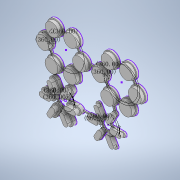
# Autodesk Inventor part: button_all
Saved by Autodesk Inventor 2022 (Build 260153000, 153)
## iProperties
Created: 2022-07-05
Part Number: button_all
Material: 常规
Document SubType Name: Modeling
Designer: yangmc
Density: 1 g/cm^3
Appearance: 默认
Author: yangmc
Autodesk Inventor part; units mm, degrees
ref_plane "YZ Plane" through (0, 0, 0) normal (1, 0, 0) x (0, 1, 0)
ref_plane "XZ Plane" through (0, 0, 0) normal (0, 1, 0) x (-1, 0, 0)
ref_plane "XY Plane" through (0, 0, 0) normal (0, 0, 1) x (1, 0, 0)
sketch "草图1" plane through (0, 0, 0) normal (0, 0, 1) x (1, 0, 0)
  line L0 (24.3527, -0.0988) -> (30.3527, -0.0988) construction
  line L1 (24.3527, -1.5988) -> (30.3527, -1.5988)
  line L2 (30.3527, 1.4012) -> (24.3527, 1.4012)
  arc A0 (24.3527, 1.4012) -> (24.3527, -1.5988) centre (24.3527, -0.0988) ccw
  arc A1 (30.3527, -1.5988) -> (30.3527, 1.4012) centre (30.3527, -0.0988) ccw
  line L3 (25.3527, -0.0988) -> (29.3527, -0.0988) construction
  line L4 (25.3527, -1.5988) -> (29.3527, -1.5988)
  line L5 (29.3527, 1.4012) -> (25.3527, 1.4012)
  arc A2 (25.3527, 1.4012) -> (25.3527, -1.5988) centre (25.3527, -0.0988) ccw
  arc A3 (29.3527, -1.5988) -> (29.3527, 1.4012) centre (29.3527, -0.0988) ccw
  circle A4 centre (-2.7903, 26.7021) radius 4.75
  circle A5 centre (-2.7903, 26.7021) radius 4
  line L6 (-3, 0) -> (3, 0) construction
  line L7 (-2, 0) -> (2, 0) construction
  line L8 (-2, -1.5) -> (2, -1.5)
  line L9 (2, 1.5) -> (-2, 1.5)
  arc A6 (-2, 1.5) -> (-2, -1.5) centre (-2, 0) ccw
  arc A7 (2, -1.5) -> (2, 1.5) centre (2, 0) ccw
  line L10 (-4.5, 0) -> (4.5, 0) construction
  line L11 (-2, -2.5) -> (2, -2.5)
  line L12 (2, 2.5) -> (-2, 2.5)
  arc A8 (-2, 2.5) -> (-2, -2.5) centre (-2, 0) ccw
  arc A9 (2, -2.5) -> (2, 2.5) centre (2, 0) ccw
  circle A10 centre (7.733, 0) radius 1.0239
  arc A11 (6.1655, -5.7149) -> (3.5674, -4.2149) centre (4.8665, -4.9649) ccw
  arc A12 (7.0315, -6.2149) -> (2.7014, -3.7149) centre (4.8665, -4.9649) ccw
  line L13 (2.8665, -8.429) -> (4.8665, -4.9649) construction
  line L14 (4.1655, -9.179) -> (6.1655, -5.7149)
  line L15 (3.5674, -4.2149) -> (1.5674, -7.679)
  line L16 (5.0315, -9.679) -> (7.0315, -6.2149)
  line L17 (2.3665, -9.295) -> (5.3665, -4.0989) construction
  line L18 (1.6165, -10.5941) -> (6.1165, -2.7998) construction
  arc A13 (1.5674, -7.679) -> (4.1655, -9.179) centre (2.8665, -8.429) ccw
  arc A14 (0.7014, -7.179) -> (5.0315, -9.679) centre (2.8665, -8.429) ccw
  line L19 (2.7014, -3.7149) -> (0.7014, -7.179)
  arc A15 (11.8985, -4.2149) -> (9.3004, -5.7149) centre (10.5994, -4.9649) ccw
  arc A16 (12.7645, -3.7149) -> (8.4344, -6.2149) centre (10.5994, -4.9649) ccw
  line L20 (12.5994, -8.429) -> (10.5994, -4.9649) construction
  line L21 (13.8985, -7.679) -> (11.8985, -4.2149)
  line L22 (9.3004, -5.7149) -> (11.3004, -9.179)
  line L23 (14.7645, -7.179) -> (12.7645, -3.7149)
  line L24 (13.0994, -9.295) -> (10.0994, -4.0989) construction
  line L25 (13.8494, -10.5941) -> (9.3494, -2.7998) construction
  arc A17 (11.3004, -9.179) -> (13.8985, -7.679) centre (12.5994, -8.429) ccw
  arc A18 (10.4344, -9.679) -> (14.7645, -7.179) centre (12.5994, -8.429) ccw
  line L26 (8.4344, -6.2149) -> (10.4344, -9.679)
  arc A19 (13.4659, 1.5) -> (13.4659, -1.5) centre (13.4659, 0) ccw
  arc A20 (13.4659, 2.5) -> (13.4659, -2.5) centre (13.4659, 0) ccw
  line L27 (17.4659, 0) -> (13.4659, 0) construction
  line L28 (17.4659, 1.5) -> (13.4659, 1.5)
  line L29 (13.4659, -1.5) -> (17.4659, -1.5)
  line L30 (17.4659, 2.5) -> (13.4659, 2.5)
  line L31 (18.4659, 0) -> (12.4659, 0) construction
  line L32 (19.9659, 0) -> (10.9659, 0) construction
  arc A21 (17.4659, -1.5) -> (17.4659, 1.5) centre (17.4659, 0) ccw
  arc A22 (17.4659, -2.5) -> (17.4659, 2.5) centre (17.4659, 0) ccw
  line L33 (13.4659, -2.5) -> (17.4659, -2.5)
  arc A23 (9.3004, 5.7149) -> (11.8985, 4.2149) centre (10.5994, 4.9649) ccw
  arc A24 (8.4344, 6.2149) -> (12.7645, 3.7149) centre (10.5994, 4.9649) ccw
  line L34 (12.5994, 8.429) -> (10.5994, 4.9649) construction
  line L35 (11.3004, 9.179) -> (9.3004, 5.7149)
  line L36 (11.8985, 4.2149) -> (13.8985, 7.679)
  line L37 (10.4344, 9.679) -> (8.4344, 6.2149)
  line L38 (13.0994, 9.295) -> (10.0994, 4.0989) construction
  line L39 (13.8494, 10.5941) -> (9.3494, 2.7998) construction
  arc A25 (13.8985, 7.679) -> (11.3004, 9.179) centre (12.5994, 8.429) ccw
  arc A26 (14.7645, 7.179) -> (10.4344, 9.679) centre (12.5994, 8.429) ccw
  line L40 (12.7645, 3.7149) -> (14.7645, 7.179)
  arc A27 (3.5674, 4.2149) -> (6.1655, 5.7149) centre (4.8665, 4.9649) ccw
  arc A28 (2.7014, 3.7149) -> (7.0315, 6.2149) centre (4.8665, 4.9649) ccw
  line L41 (2.8665, 8.429) -> (4.8665, 4.9649) construction
  line L42 (1.5674, 7.679) -> (3.5674, 4.2149)
  line L43 (6.1655, 5.7149) -> (4.1655, 9.179)
  line L44 (0.7014, 7.179) -> (2.7014, 3.7149)
  line L45 (2.3665, 9.295) -> (5.3665, 4.0989) construction
  line L46 (1.6165, 10.5941) -> (6.1165, 2.7998) construction
  arc A29 (4.1655, 9.179) -> (1.5674, 7.679) centre (2.8665, 8.429) ccw
  arc A30 (5.0315, 9.679) -> (0.7014, 7.179) centre (2.8665, 8.429) ccw
  line L47 (7.0315, 6.2149) -> (5.0315, 9.679)
  line L48 (5.3165, 2.5057) -> (4.3434, 0.8709)
  line L49 (3.8438, 1.6883) -> (4.3886, 2.511)
  line L50 (4.3263, -2.5239) -> (3.8862, -1.6408)
  line L51 (4.3547, -0.8399) -> (5.284, -2.5)
  line L52 (8.2154, -4.2122) -> (7.2306, -4.1518)
  line L53 (6.7712, -3.3456) -> (8.6735, -3.3709)
  line L54 (11.6221, -1.6883) -> (11.0773, -2.511)
  line L55 (10.1494, -2.5057) -> (11.1225, -0.8709)
  line L56 (11.1396, 2.5239) -> (11.5797, 1.6408)
  line L57 (11.1112, 0.8399) -> (10.1819, 2.5)
  line L58 (7.2505, 4.2122) -> (8.2354, 4.1518)
  line L59 (8.6947, 3.3456) -> (6.7924, 3.3709)
  line L60 (22.5273, 0) -> (28.5273, 0) construction
  line L61 (21.0273, 0) -> (30.0273, 0) construction
  circle A31 centre (2.7186, 16.9267) radius 4.75
  circle A32 centre (2.7186, 16.9267) radius 4
  circle A33 centre (13.9389, 16.8098) radius 4.75
  circle A34 centre (13.9389, 16.8098) radius 4
  circle A35 centre (19.6501, 26.4684) radius 4.75
  circle A36 centre (19.6501, 26.4684) radius 4
  circle A37 centre (14.1412, 36.2438) radius 4.75
  circle A38 centre (14.1412, 36.2438) radius 4
  circle A39 centre (2.921, 36.3607) radius 4.75
  circle A40 centre (2.921, 36.3607) radius 4
  line L62 (0.3592, 32.3607) -> (-0.5039, 30.8656)
  line L63 (0.6205, 31.2131) -> (1.0674, 31.9872)
  line L64 (0.6205, 31.2131) -> (0.1636, 30.4218)
  line L65 (-0.6071, 22.4835) -> (0.2561, 20.9885)
  line L66 (0.5173, 22.136) -> (0.9742, 21.3447)
  line L67 (0.5173, 22.136) -> (0.0704, 22.9101)
  line L68 (7.4636, 16.7081) -> (9.19, 16.7081)
  line L69 (8.3268, 17.5081) -> (9.2405, 17.5081)
  line L70 (8.3268, 17.5081) -> (7.4329, 17.5081)
  line L71 (16.5006, 20.8098) -> (17.3638, 22.3049)
  line L72 (16.2394, 21.9574) -> (16.6962, 22.7486)
  line L73 (16.2394, 21.9574) -> (15.7924, 21.1832)
  line L74 (17.4669, 30.687) -> (16.6037, 32.182)
  line L75 (16.3425, 31.0345) -> (15.8857, 31.8258)
  line L76 (16.3425, 31.0345) -> (16.7894, 30.2604)
  line L77 (9.3962, 36.4624) -> (7.6699, 36.4624)
  line L78 (8.5331, 35.6624) -> (7.6194, 35.6624)
  line L79 (8.5331, 35.6624) -> (9.4269, 35.6624)
  circle A41 centre (31.494, 26.7021) radius 4.75
  circle A42 centre (31.494, 26.7021) radius 4
  circle A43 centre (37.003, 16.9267) radius 4.75
  circle A44 centre (37.003, 16.9267) radius 4
  circle A45 centre (48.2232, 16.8098) radius 4.75
  circle A46 centre (48.2232, 16.8098) radius 4
  circle A47 centre (53.9345, 26.4684) radius 4.75
  circle A48 centre (53.9345, 26.4684) radius 4
  circle A49 centre (48.4255, 36.2438) radius 4.75
  circle A50 centre (48.4255, 36.2438) radius 4
  circle A51 centre (37.2053, 36.3607) radius 4.75
  circle A52 centre (37.2053, 36.3607) radius 4
  line L80 (34.6436, 32.3606) -> (33.7804, 30.8656)
  line L81 (34.9048, 31.2131) -> (35.3517, 31.9872)
  line L82 (34.9048, 31.2131) -> (34.448, 30.4218)
  line L83 (33.6773, 22.4835) -> (34.5404, 20.9885)
  line L84 (34.8017, 22.136) -> (35.2585, 21.3447)
  line L85 (34.8017, 22.136) -> (34.3547, 22.9101)
  line L86 (41.7479, 16.7081) -> (43.4743, 16.7081)
  line L87 (42.6111, 17.5081) -> (43.5248, 17.5081)
  line L88 (42.6111, 17.5081) -> (41.7172, 17.5081)
  line L89 (50.7849, 20.8098) -> (51.6481, 22.3049)
  line L90 (50.5237, 21.9574) -> (50.9805, 22.7486)
  line L91 (50.5237, 21.9574) -> (50.0768, 21.1833)
  line L92 (51.7512, 30.687) -> (50.8881, 32.182)
  line L93 (50.6268, 31.0345) -> (50.17, 31.8258)
  line L94 (50.6268, 31.0345) -> (51.0738, 30.2604)
  line L95 (43.6806, 36.4624) -> (41.9542, 36.4624)
  line L96 (42.8174, 35.6624) -> (41.9037, 35.6624)
  line L97 (42.8174, 35.6624) -> (43.7112, 35.6624)
  line L98 (24.4001, 26.4684) -> (26.7498, 26.4684)
  line L99 (24.2834, 27.5149) -> (26.8141, 27.5149)
  line L100 (31.1148, -2.8629) -> (28.1148, -8.0591)
  line L101 (30.6148, -3.729) -> (28.6148, -7.1931)
  line L102 (29.4139, -8.8091) -> (32.4139, -3.6129) construction
  line L103 (29.9139, -7.9431) -> (31.9139, -4.479) construction
  arc A53 (33.7129, -4.3629) -> (31.1148, -2.8629) centre (32.4139, -3.6129) ccw
  arc A54 (33.2129, -5.229) -> (30.6148, -3.729) centre (31.9139, -4.479) ccw
  line L104 (30.7129, -9.5591) -> (33.7129, -4.3629)
  arc A55 (28.6148, -7.1931) -> (31.2129, -8.6931) centre (29.9139, -7.9431) ccw
  arc A56 (28.1148, -8.0591) -> (30.7129, -9.5591) centre (29.4139, -8.8091) ccw
  line L105 (31.2129, -8.6931) -> (33.2129, -5.229)
  line L106 (35.1887, -4.335) -> (38.1887, -9.5312)
  line L107 (35.6887, -5.201) -> (37.6887, -8.6651)
  line L108 (39.4877, -8.7812) -> (36.4877, -3.585) construction
  line L109 (38.9877, -7.9151) -> (36.9877, -4.451) construction
  arc A57 (37.7868, -2.835) -> (35.1887, -4.335) centre (36.4877, -3.585) ccw
  arc A58 (38.2868, -3.701) -> (35.6887, -5.201) centre (36.9877, -4.451) ccw
  line L110 (40.7868, -8.0312) -> (37.7868, -2.835)
  arc A59 (37.6887, -8.6651) -> (40.2868, -7.1651) centre (38.9877, -7.9151) ccw
  arc A60 (38.1887, -9.5312) -> (40.7868, -8.0312) centre (39.4877, -8.7812) ccw
  line L111 (40.2868, -7.1651) -> (38.2868, -3.701)
  line L112 (38.5005, -1.543) -> (44.5005, -1.543)
  line L113 (39.5005, -1.543) -> (43.5005, -1.543)
  line L114 (44.5005, -0.043) -> (38.5005, -0.043) construction
  line L115 (43.5005, -0.043) -> (39.5005, -0.043) construction
  arc A61 (38.5005, 1.457) -> (38.5005, -1.543) centre (38.5005, -0.043) ccw
  arc A62 (39.5005, 1.457) -> (39.5005, -1.543) centre (39.5005, -0.043) ccw
  line L116 (44.5005, 1.457) -> (38.5005, 1.457)
  arc A63 (43.5005, -1.543) -> (43.5005, 1.457) centre (43.5005, -0.043) ccw
  arc A64 (44.5005, -1.543) -> (44.5005, 1.457) centre (44.5005, -0.043) ccw
  line L117 (43.5005, 1.457) -> (39.5005, 1.457)
  line L118 (37.7384, 2.7211) -> (40.7384, 7.9173)
  line L119 (38.2384, 3.5872) -> (40.2384, 7.0513)
  line L120 (39.4393, 8.6673) -> (36.4393, 3.4711) construction
  line L121 (38.9393, 7.8013) -> (36.9393, 4.3372) construction
  arc A65 (35.1403, 4.2211) -> (37.7384, 2.7211) centre (36.4393, 3.4711) ccw
  arc A66 (35.6403, 5.0872) -> (38.2384, 3.5872) centre (36.9393, 4.3372) ccw
  line L122 (38.1403, 9.4173) -> (35.1403, 4.2211)
  arc A67 (40.2384, 7.0513) -> (37.6403, 8.5513) centre (38.9393, 7.8013) ccw
  arc A68 (40.7384, 7.9173) -> (38.1403, 9.4173) centre (39.4393, 8.6673) ccw
  line L123 (37.6403, 8.5513) -> (35.6403, 5.0872)
  line L124 (33.6645, 4.1932) -> (30.6645, 9.3894)
  line L125 (33.1645, 5.0592) -> (31.1645, 8.5233)
  line L126 (29.3655, 8.6394) -> (32.3655, 3.4432) construction
  line L127 (29.8655, 7.7733) -> (31.8655, 4.3092) construction
  arc A69 (31.0664, 2.6932) -> (33.6645, 4.1932) centre (32.3655, 3.4432) ccw
  arc A70 (30.5664, 3.5592) -> (33.1645, 5.0592) centre (31.8655, 4.3092) ccw
  line L128 (28.0664, 7.8894) -> (31.0664, 2.6932)
  arc A71 (31.1645, 8.5233) -> (28.5664, 7.0233) centre (29.8655, 7.7733) ccw
  arc A72 (30.6645, 9.3894) -> (28.0664, 7.8894) centre (29.3655, 8.6394) ccw
  line L129 (28.5664, 7.0233) -> (30.5664, 3.5592)
  line L130 (31.1645, 1.1625) -> (31.6155, 2.1442)
  line L131 (32.6639, 1.9732) -> (31.8304, 0.1589)
  line L132 (31.7274, -2.2792) -> (31.1027, -1.3979)
  line L133 (31.775, -0.5754) -> (32.9295, -2.2043)
  line L134 (34.9895, -3.5127) -> (33.9139, -3.6129)
  line L135 (33.5377, -2.6195) -> (35.5256, -2.4342)
  line L136 (37.6887, -1.3043) -> (37.2377, -2.286)
  line L137 (36.1893, -2.115) -> (37.0228, -0.3008)
  line L138 (37.1258, 2.1374) -> (37.7505, 1.2561)
  line L139 (37.0782, 0.4336) -> (35.9238, 2.0625)
  line L140 (33.8637, 3.3709) -> (34.9393, 3.4711)
  line L141 (35.3155, 2.4777) -> (33.3276, 2.2924)
  line L142 (2.8665, 10.929) -> (2.8665, 12.179)
  line L143 (2.0184, 12.2285) -> (2.0184, 10.7808)
  line L144 (38.9393, 12.5893) -> (39.7377, 10.1373)
  line L145 (37.7032, 12.2285) -> (38.4858, 9.8252)
  line L146 (19.9659, 0) -> (22.856, 0)
  line L147 (19.8206, 0.8399) -> (23.1828, 0.8399)
  point P0 (0, 0)
  point P1 (27.3527, -0.0988)
  point P2 (8.549, -2.2811)
  point P3 (5.951, -3.7811)
  point P4 (7.951, -7.2452)
  point P5 (10.549, -5.7452)
  point P6 (5.951, 3.7811)
  point P7 (8.549, 2.2811)
  point P8 (10.549, 5.7452)
  point P9 (7.951, 7.2452)
  point P10 (0, 0)
  point P11 (0, 0)
  point P12 (4.3547, 0.8399)
  point P13 (4.3547, -0.8399)
  point P14 (5.3165, -2.5057)
  point P15 (6.7712, -3.3456)
  point P16 (3.8665, -6.6969)
  point P17 (8.6947, -3.3456)
  point P18 (10.1494, -2.5057)
  point P19 (11.5994, -6.6969)
  point P20 (11.1112, -0.8399)
  point P21 (11.1112, 0.8399)
  point P22 (15.4659, 0)
  point P23 (10.1494, 2.5057)
  point P24 (8.6947, 3.3456)
  point P25 (11.5994, 6.6969)
  point P26 (6.7712, 3.3456)
  point P27 (3.8665, 6.6969)
  point P28 (11.1225, -0.8709)
  point P29 (32.7578, -4.1518)
  point P30 (33.7427, -4.2122)
  point P31 (34.2008, -3.3709)
  point P32 (32.2985, -3.3456)
  point P33 (35.6767, -2.5057)
  point P34 (36.6046, -2.511)
  point P35 (37.1494, -1.6883)
  point P36 (36.6498, -0.8709)
  point P37 (36.6385, 0.8399)
  point P38 (37.107, 1.6408)
  point P39 (36.6669, 2.5239)
  point P40 (35.7092, 2.5)
  point P41 (32.7778, 4.2122)
  point P42 (32.3197, 3.3709)
  point P43 (34.222, 3.3456)
  point P44 (33.7627, 4.1518)
  point P45 (29.8536, -2.5239)
  point P46 (30.8113, -2.5)
  point P47 (29.882, -0.8399)
  point P48 (29.4135, -1.6408)
  point P49 (8.6735, -26.4255)
  point P50 (6.7712, -26.4003)
  point P51 (7.2306, -27.2064)
  point P52 (8.2154, -27.2669)
  point P53 (4.3263, -25.5786)
  point P54 (5.284, -25.5547)
  point P55 (4.3547, -23.8945)
  point P56 (3.8862, -24.6954)
  point P57 (7.2505, -18.8424)
  point P58 (6.7924, -19.6838)
  point P59 (8.6947, -19.7091)
  point P60 (8.2354, -18.9029)
  point P61 (10.1819, -20.5547)
  point P62 (11.1112, -22.2148)
  point P63 (11.5797, -21.4139)
  point P64 (11.1396, -20.5307)
  point P65 (11.1225, -23.9255)
  point P66 (10.1494, -25.5604)
  point P67 (11.0773, -25.5656)
  point P68 (11.6221, -24.743)
  point P69 (13.8494, -12.4606)
  point P70 (13.8494, -10.5941)
  point P71 (1.6165, -12.4606)
  point P72 (8.4299, 26.5852)
  point P73 (8.4299, 26.5852)
  point P74 (42.7142, 26.5852)
  point P75 (42.7142, 26.5852)
  point P76 (34.4266, -0.0709)
  point P77 (30.9139, -6.211)
  point P78 (37.9877, -6.1831)
  point P79 (41.5005, -0.043)
  point P80 (37.9393, 6.0692)
  point P81 (30.8655, 6.0413)
  point P82 (28.5664, 7.0233)
  point P83 (30.5664, 3.5592)
  point P84 (37.6403, 8.5513)
  point P85 (35.6403, 5.0872)
  point P86 (43.5005, 1.457)
  point P87 (39.5005, 1.457)
  point P88 (40.2868, -7.1651)
  point P89 (38.2868, -3.701)
  point P90 (31.2129, -8.6931)
  point P91 (33.2129, -5.229)
  point P92 (11.1225, -0.8709)
  dimension "d2" = 3
  dimension "d3" = 3
  dimension "d4" = 2
  dimension "d5" = 3
  dimension "d7" = 9.5
  dimension "d8" = 8
  dimension "d27" = 3
  dimension "d28" = 2
  dimension "d29" = 3
  dimension "d30" = 9
  dimension "d31" = 5
  dimension "d32" = 360
  dimension "d33" = 360
  dimension "d46" = 360
  dimension "d51" = 360
  dimension "d61" = 9.5
  dimension "d62" = 8
  dimension "d63" = 360
  dimension "d64" = 360
  dimension "d67" = 360
  dimension "d71" = 360
  constraints: 360 end point, 150 point on circle, 73 centre point, 43 point on line, 26 coincident, 16 tangent, 8 parallel, 5 midpoint, 4 horizontal, 2 vertical, 554 other
  measures "d2" distance of point (27.353, -0.099) L0.end
  measures "d3" diameter of A1
  measures "d4" distance of point (27.353, -0.099) L3.end
  measures "d5" diameter of A3
  measures "d7" diameter of A4
  measures "d8" diameter of A5
  measures "d27" distance of point (0, 0) L6.end
  measures "d28" distance of point (0, 0) L7.end
  measures "d29" diameter of A7
  measures "d30" distance of L10.start L10.end
  measures "d31" diameter of A9
  measures "d61" diameter of A41
  measures "d62" diameter of A42
extrude "拉伸1" add sketch "草图1" along normal blind 1.2 contours A31 | A43 | A33 | A41 | A4 | A45 | A35 | A39 | A47 | A51 | A37 | A49
extrude "拉伸2" add sketch "草图1" along normal blind 3.2 contours A5 | A32 | A34 | A36 | A38 | A40 | A42 | A44 | A46 | A48 | A50 | A52
extrude "拉伸3" add sketch "草图1" along normal blind 2.2 contours A22 L33 A20 L30 | A16 L23 A18 L26 | A24 L37 A26 L40 | A12 L16 A14 L19 | A28 L44 A30 L47 | A9 L11 A8 L12
extrude "拉伸4" add sketch "草图1" along normal blind 4.7 contours A6 L9 A7 L8 | L14 A13 L15 A11 | L21 A17 L22 A15 | L28 A21 L29 A19 | L35 A25 L36 A23 | L42 A29 L43 A27
extrude "拉伸5" add sketch "草图1" along normal blind 2.8 contours A2 L2 A3 L1 | A54 L104 A55 L100 | L128 A71 L124 A70 | A58 L110 A59 L106 | L122 A67 L118 A66 | A62 L116 A63 L112
extrude "拉伸6" add sketch "草图1" along normal blind 1 contours A0 L2 A2 L1 | A3 L2 A1 L1 | A53 L104 A54 L100 | A69 L128 A70 L124 | A57 L110 A58 L106 | A55 L104 A56 L100 | A65 L122 A66 L118 | L128 A72 L124 A71 | A61 L116 A62 L112 | A59 L110 A60 L106 | L122 A68 L118 A67 | A63 L116 A64 L112
extrude "拉伸7" add sketch "草图1" along normal blind 0.8 contours L146 A22 L147 A0 | A1 L133 A53 L132 | L130 A69 L131 A1 | L54 A16 L55 A20 | A20 L57 A24 L56 | L135 A57 L134 A53 | A69 L140 A65 L141 | A16 L52 A12 L53 | L137 A61 L136 A57 | L59 A28 L58 A24 | A65 L138 A61 L139 | A12 L50 A9 L51 | L48 A9 L49 A28 | A30 L143 A31 L142 | L145 A43 L144 A68 | A31 L70 L69 A33 L68 | L83 A41 L85 L84 A43 | L65 A4 L67 L66 A31 | A43 L88 L87 A45 L86 | L98 A35 L99 A41 | L62 A39 L63 L64 A4 | L73 L72 A35 L71 A33 | L91 L90 A47 L89 A45 | L80 A51 L81 L82 A41 | L77 A37 L79 L78 A39 | A35 L76 L75 A37 L74 | L95 A49 L97 L96 A51 | L94 L93 A49 L92 A47
